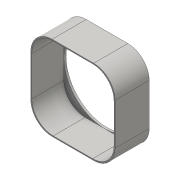
# Autodesk Inventor part: Motor mount (plain)
Saved by Autodesk Inventor 2016 (Build 200138000, 138)
## iProperties
Created: 2016-03-10
Part Number: Motor mount (plain)
Material: Generic
Document SubType Name: Modeling
Designer: s_sud
Density: 1 g/cm^3
Appearance: Default
Author: s_sud
Autodesk Inventor part; units mm, degrees
ref_plane "YZ Plane" through (0, 0, 0) normal (1, 0, 0) x (0, 1, 0)
ref_plane "XZ Plane" through (0, 0, 0) normal (0, 1, 0) x (-1, 0, 0)
ref_plane "XY Plane" through (0, 0, 0) normal (0, 0, 1) x (1, 0, 0)
sketch "Sketch1" plane through (0, 0, 0) normal (0, 1, 0) x (-1, 0, 0)
  circle A0 centre (0, 0) radius 38.5
  circle A1 centre (0, 0) radius 39.5
  dimension "d0" = 77
  dimension "d1" = 79
  constraints: 2 centre point, 2 coincident
  measures "d0" diameter of A0
  measures "d1" diameter of A1
extrude "Extrusion1" add sketch "Sketch1" along normal blind 2
sketch "Sketch21" plane through (0, 2, 0) normal (0, 1, 0) x (1, 0, 0)
  line L0 (-39.5, -39.5) -> (39.5, -39.5)
  line L1 (39.5, -39.5) -> (39.5, 39.5)
  line L2 (39.5, 39.5) -> (-39.5, 39.5)
  line L3 (-39.5, 39.5) -> (-39.5, -39.5)
  line L4 (-39.5, -39.5) -> (39.5, 39.5) construction
  line L5 (39.5, -39.5) -> (-39.5, 39.5) construction
  circle A0 centre (0, 0) radius 39.5
  dimension "d111" = 79
  dimension "d112" = 79
  constraints: 12 end point, 2 midpoint, 2 parallel, 1 centre point, 1 coincident, 1 horizontal, 1 perpendicular, 1 tangent
  measures "d111" distance of L2.end L0.start
  measures "d112" distance of L0.start L0.end
extrude "Extrusion21" add sketch "Sketch21" against normal blind 2 contours L3 A0 L0 | A0 L1 L0 | L3 L2 A0 | A0 L2 L1
fillet "Fillet3" radius 20 4 edges at (-39.5, 1, -39.5) (39.5, 1, -39.5) (39.5, 1, 39.5) (-39.5, 1, 39.5)
sketch "Sketch24" plane through (0, 0, 0) normal (0, -1, 0) x (1, 0, 0)
  arc A0 (-19.5, 39.5) -> (-39.5, 19.5) centre (-19.5, 19.5) ccw projected
  circle A1 centre (0, 0) radius 38.5 projected
  arc A2 (-19.5, 39.5) -> (-39.5, 19.5) centre (-19.5, 19.5) ccw projected
  line L0 (-39.5, 19.5) -> (-39.5, -19.5) projected
  arc A3 (-39.5, -19.5) -> (-19.5, -39.5) centre (-19.5, -19.5) ccw projected
  line L1 (-19.5, -39.5) -> (19.5, -39.5) projected
  arc A4 (19.5, -39.5) -> (39.5, -19.5) centre (19.5, -19.5) ccw projected
  line L2 (39.5, -19.5) -> (39.5, 19.5) projected
  arc A5 (39.5, 19.5) -> (19.5, 39.5) centre (19.5, 19.5) ccw projected
  line L3 (19.5, 39.5) -> (-19.5, 39.5) projected
  line L4 (-18.5, -38.5) -> (18.5, -38.5)
  line L5 (38.5, -18.5) -> (38.5, 18.5)
  line L6 (18.5, 38.5) -> (-18.5, 38.5)
  line L7 (-38.5, 18.5) -> (-38.5, -18.5)
  line L8 (-38.5, -38.5) -> (38.5, 38.5) construction
  line L9 (38.5, -38.5) -> (-38.5, 38.5) construction
  arc A6 (-36.5, 38.5) -> (-38.5, 36.5) centre (-36.5, 36.5) ccw
  arc A7 (38.5, 18.5) -> (18.5, 38.5) centre (18.5, 18.5) ccw
  arc A8 (-18.5, 38.5) -> (-38.5, 18.5) centre (-18.5, 18.5) ccw
  arc A9 (-38.5, -18.5) -> (-18.5, -38.5) centre (-18.5, -18.5) ccw
  arc A10 (18.5, -38.5) -> (38.5, -18.5) centre (18.5, -18.5) ccw
  dimension "d133" = 77
  dimension "d134" = 77
  dimension "d135" = 2
  dimension "d136" = 20
  constraints: 12 end point, 10 point on circle, 10 point on line, 10 tangent, 5 centre point, 3 equal radius, 2 midpoint, 2 parallel, 1 horizontal, 1 perpendicular
  measures "d133" distance of L9.end L8.end
  measures "d134" distance of L9.start L8.end
  measures "d135" radius of A6
  measures "d136" radius of A7
extrude "Extrusion24" add sketch "Sketch24" along normal blind 30
body "Solid1"
